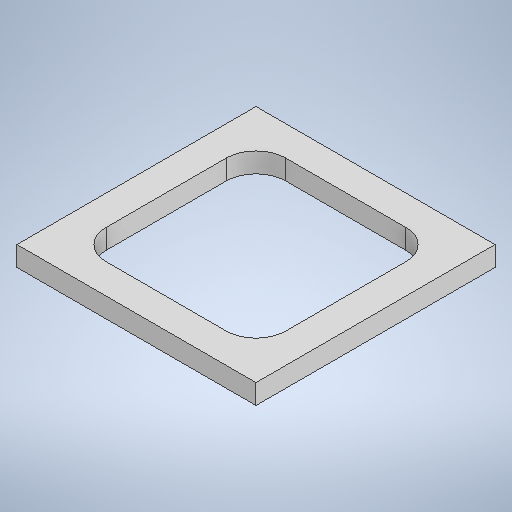
# Autodesk Inventor part: mould
Saved by Autodesk Inventor 2025.3 (Build 293356030, 356C)
## iProperties
Created: 2025-09-03
Part Number: mould
Material: Generic
Document SubType Name: Sheet Metal
Designer: robert
Density: 1 g/cm^3
Sheet Metal Rule: Default_mm
Appearance: Default
Author: robert
Autodesk Inventor part; units mm, degrees
ref_plane "YZ Plane" through (0, 0, 0) normal (1, 0, 0) x (0, 1, 0)
ref_plane "XZ Plane" through (0, 0, 0) normal (0, 1, 0) x (-1, 0, 0)
ref_plane "XY Plane" through (0, 0, 0) normal (0, 0, 1) x (1, 0, 0)
sketch "Sketch2" plane through (0, 0, 0) normal (0, 1, 0) x (-1, 0, 0)
  line L0 (-22, 59.152) -> (-34, 59.152)
  arc A0 (-34, 59.152) -> (-35.5236, 58.7363) centre (-34, 56.152) ccw
  arc A1 (-35.5236, 58.7363) -> (-36.5843, 57.6756) centre (-34, 56.152) ccw
  arc A2 (-36.5843, 57.6756) -> (-37, 56.152) centre (-34, 56.152) ccw
  line L1 (-37, 56.152) -> (-37, 44.152)
  arc A3 (-37, 44.052) -> (-34, 41.052) centre (-34, 44.052) ccw
  line L2 (-33.9, 41.052) -> (-21.9, 41.052)
  arc A4 (-21.9, 41.052) -> (-18.9, 44.052) centre (-21.9, 44.052) ccw
  line L3 (-18.9, 44.152) -> (-18.9, 56.152)
  arc A5 (-18.9, 56.152) -> (-21.9, 59.152) centre (-21.9, 56.152) ccw
  line L4 (-15.9, 62.152) -> (-40, 62.152)
  line L5 (-40, 62.152) -> (-40, 38.052)
  line L6 (-40, 38.052) -> (-15.9, 38.052)
  line L7 (-15.9, 38.052) -> (-15.9, 62.152)
  line L8 (-21.9, 59.152) -> (-22, 59.152)
  line L9 (-37, 44.152) -> (-37, 44.052)
  line L10 (-33.9, 41.052) -> (-34, 41.052)
  line L11 (-18.9, 44.152) -> (-18.9, 44.052)
  point P0 (0, 0)
  dimension "d6" = 18.1
  dimension "d7" = 18.1
  dimension "d14" = 3
  dimension "d24" = 3
  dimension "d25" = 3
  dimension "d28" = 3
  dimension "d29" = 3
  constraints: 24 end point, 13 point on circle, 6 centre point, 2 parallel, 2 perpendicular, 1 collinear, 1 horizontal, 1 tangent, 1 vertical
  measures "d6" distance between parallel lines of L1 L3
  measures "d7" distance between parallel lines of L0 L2
  measures "d14" radius of A4
  measures "d24" distance between parallel lines of L4 L0
  measures "d25" distance between parallel lines of L1 L5
  measures "d28" distance between parallel lines of L7 L3
  measures "d29" distance between parallel lines of L2 L6
extrude "Extrusion1" add sketch "Sketch2" along normal blind 2
equation "\"BendRadius\" = Thickness"
equation "\"BendReliefWidth\" = Thickness"
equation "\"BendReliefDepth\" = 0.5 * Thickness"
equation "\"CornerReliefSize\" = 4 * Thickness"
equation "\"MinimumRemnant\" = 2 * Thickness"
equation "\"TransitionRadius\" = BendRadius"
equation "\"JacobiRadiusSize\" = BendRadius"
equation "\"GapSize\" = Thickness"
equation "\"Thickness\" = 0.5"
body "Solid1"
